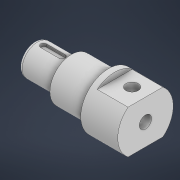
# Autodesk Inventor part: Pieza de practica 11
Saved by Autodesk Inventor 2022 (Build 260153000, 153)
## iProperties
Created: 2022-08-24
Part Number: Pieza de practica 11
Material: Genérico
Document SubType Name: Modeling
Designer: aleon
Density: 1 g/cm^3
Appearance: Valor por defecto
Author: aleon
Autodesk Inventor part; units mm, degrees
ref_plane "YZ Plane" through (0, 0, 0) normal (1, 0, 0) x (0, 1, 0)
ref_plane "XY Plane" through (0, 0, 0) normal (0, 0, 1) x (1, 0, 0)
sketch "Boceto1" plane through (0, 0, 0) normal (0, 1, 0) x (-1, 0, 0)
  line L0 (0, 0) -> (72, 0)
  line L1 (72, 0) -> (72, 10)
  line L2 (72, 10) -> (48, 10)
  line L3 (48, 10) -> (48, 14)
  line L4 (48, 14) -> (24, 14)
  line L5 (24, 14) -> (24, 18)
  line L6 (24, 18) -> (0, 18)
  line L7 (0, 18) -> (0, 0)
  dimension "d15" = 72
  dimension "d16" = 10
  dimension "d17" = 24
  dimension "d18" = 4
  dimension "d19" = 24
  dimension "d20" = 4
  constraints: 16 end point, 6 perpendicular, 1 horizontal, 1 vertical
  measures "d15" distance of L0.start L0.end
  measures "d16" distance of L0.end L1.end
  measures "d17" distance of L1.end L2.end
  measures "d18" distance of L2.end L3.end
  measures "d19" distance of L3.end L4.end
  measures "d20" distance of L4.end L5.end
revolve "Revolución2" add sketch "Boceto1" angle 360 about axis through (0, 0, 0) along (-1, 0, 0)
sketch "Boceto2" plane through (0, 0, 0) normal (1, 0, 0) x (0, 0, -1)
  line L0 (-11.3137, 14) -> (11.3137, 14)
  circle A0 centre (0, 0) radius 18 projected
  line L1 (-11.3137, -14) -> (11.3137, -14)
  dimension "d22" = 14
  dimension "d25" = 14
  constraints: 4 end point, 4 point on circle, 2 horizontal
  measures "d22" distance from line of L0 point (0, 0)
  measures "d25" distance from line of L1 point (0, 0)
extrude "Extrusión1" cut sketch "Boceto2" against normal blind 20 contours A0 L0 | L1 A0
sketch "Boceto3" plane through (0, 14, 11.3137) normal (0, 1, 0) x (1, 0, 0)
  circle A0 centre (-10, 12.6274) radius 4
  line L0 (-20, 22.6274) -> (0, 22.6274) projected
  line L1 (0, 22.6274) -> (0, 0) projected
  point P0 (0, 11.3137)
  dimension "d26" = 8
  dimension "d28" = 10
  dimension "d29" = 10
  constraints: 1 centre point
  measures "d26" diameter of A0
  measures "d28" distance from line of L0 A0.centre
  measures "d29" distance from line of L1 A0.centre
extrude "Extrusión2" cut sketch "Boceto3" against normal through all
sketch "Boceto4" plane through (0, 0, 0) normal (1, 0, 0) x (0, 0, -1)
  circle A0 centre (0, 0) radius 4
  dimension "d32" = 8
  constraints: 1 centre point, 1 coincident
  measures "d32" diameter of A0
extrude "Extrusión3" cut sketch "Boceto4" against normal through all
fillet "Empalme1" radius 2 1 edges at (-72, 0, -10)
ref_plane "Plano de trabajo1" through (0, 10, 0) normal (0, 1, 0) x (-1, 0, 0)
sketch "Boceto5" plane through (0, 10, 0) normal (0, 1, 0) x (-1, 0, 0)
  line L0 (54, 2) -> (66, 2)
  line L1 (68, 0) -> (68, 0)
  line L2 (66, -2) -> (54, -2)
  line L3 (52, 0) -> (52, 0)
  line L4 (52, 2) -> (68, -2) construction
  line L5 (68, 2) -> (52, -2) construction
  arc A0 (68, 0) -> (66, 2) centre (66, 0) ccw
  arc A1 (66, -2) -> (68, 0) centre (66, 0) ccw
  arc A2 (54, 2) -> (52, 0) centre (54, 0) ccw
  arc A3 (52, 0) -> (54, -2) centre (54, 0) ccw
  line L6 (48, -14) -> (48, 14) projected
  point P0 (0, 0)
  point P1 (60, 0)
  point P2 (52, 0)
  point P3 (68, 0)
  dimension "d37" = 16
  dimension "d38" = 4
  dimension "d39" = 2
  dimension "d40" = 12
  constraints: 12 end point, 8 point on circle, 8 point on line, 8 tangent, 4 centre point, 3 equal radius, 2 midpoint, 2 parallel, 1 horizontal, 1 perpendicular
  measures "d37" distance of L4.end L5.end
  measures "d38" distance of L5.start L4.end
  measures "d39" radius of A0
  measures "d40" distance from line of L6 point (60, 0)
extrude "Extrusión4" cut sketch "Boceto5" against normal blind 2
mirror "Simetría1" about plane through (0, 0, 0) normal (0, 1, 0) of "Extrusión4"
